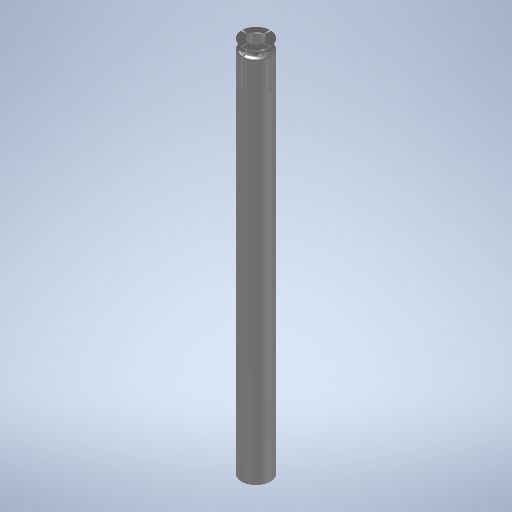
# Autodesk Inventor part: specimen_holder_rod_6mm
Saved by Autodesk Inventor 2023.2 (Build 272271000, 271)
## iProperties
Created: 2015-09-24
Part Number: specimen_holder_rod_6mm
Material: Edelstahl
Document SubType Name: Modeling
Designer: splath
Density: 8.08 g/cm^3
Appearance: Halbpoliert
Mass: 9.27092 g
Surface Area: 14.4867 cm^2
Volume: 1.14739 cm^3
Author: splath
Autodesk Inventor part; units mm, degrees
ref_plane "YZ Plane" through (0, 0, 0) normal (1, 0, 0) x (0, 1, 0)
ref_plane "XZ Plane" through (0, 0, 0) normal (0, 1, 0) x (-1, 0, 0)
sketch "Skizze1" plane through (0, 0, 0) normal (0, 0, 1) x (1, 0, 0)
  circle A0 centre (0, 0) radius 3
  dimension "d2" = 6
  constraints: 1 centre point, 1 coincident
  measures "d2" diameter of A0
extrude "Extrusion1" add sketch "Skizze1" against normal blind 70
sketch "Skizze2" plane through (0, 0, 0) normal (0, 0, 1) x (1, 0, 0)
  circle A0 centre (0, 0) radius 3 projected
  circle A1 centre (0, 0) radius 3
  dimension "d36" = 6
  constraints: 1 centre point, 1 coincident
  measures "d36" diameter of A1
extrude "Extrusion2" add sketch "Skizze2" along normal blind 1
sketch "Skizze3" plane through (0, 0, 1) normal (0, 0, 1) x (1, 0, 0)
  circle A0 centre (0, 0) radius 3 projected
  circle A1 centre (0, 0) radius 3
  dimension "d28" = 6
  constraints: 1 centre point, 1 coincident
  measures "d28" diameter of A1
extrude "Extrusion3" add sketch "Skizze3" along normal blind 8
ref_plane "Arbeitsebene1" through (0, 0, 2.5) normal (0, 0, 1) x (1, 0, 0)
sketch "Skizze4" plane through (0, 0, 2.5) normal (0, 0, 1) x (1, 0, 0)
  circle A0 centre (0, 0) radius 3
  constraints: 1 centre point, 1 coincident
extrude "Extrusion4" [suppressed]
hole "Bohrung1" at (0, 0, 9) direction (0, 0, -1) diameter 3 depth 23
chamfer "Fase1" distance 0.1 angle 45 1 edges at (0, 1.5, 9)
sketch "Skizze5" plane through (0, 0, 9) normal (0, 0, 1) x (1, 0, 0)
  circle A0 centre (0, 0) radius 3 projected
  line L0 (-3.5, -0.15) -> (3.5, -0.15)
  line L1 (3.5, -0.15) -> (3.5, 0.15)
  line L2 (3.5, 0.15) -> (-3.5, 0.15)
  line L3 (-3.5, 0.15) -> (-3.5, -0.15)
  line L4 (-3.5, -0.15) -> (3.5, 0.15) construction
  line L5 (3.5, -0.15) -> (-3.5, 0.15) construction
  line L6 (-0.15, -3.5) -> (0.15, -3.5)
  line L7 (0.15, -3.5) -> (0.15, 3.5)
  line L8 (0.15, 3.5) -> (-0.15, 3.5)
  line L9 (-0.15, 3.5) -> (-0.15, -3.5)
  line L10 (-0.15, -3.5) -> (0.15, 3.5) construction
  line L11 (0.15, -3.5) -> (-0.15, 3.5) construction
  constraints: 24 end point, 4 midpoint
extrude "Extrusion5" cut sketch "Skizze5" against normal up to surface (8 mm away) contours A0 L0 L7 L2 | A0 L2 L1 L0 | L7 L2 L9 A0 | A0 L9 L8 L7 | L7 L0 L9 L2 | L7 L6 L9 A0 | A0 L9 L0 L7 | L9 L0 A0 L2 | A0 L0 L3 L2
sketch "Skizze6" plane through (0, 0, 0) normal (0, 1, 0) x (-1, 0, 0)
  line L0 (0, 0) -> (-2, 0)
  line L1 (0, -1.8) -> (0, 10.8) projected
  circle A0 centre (-3, 8) radius 1
  line L2 (-0.15, 9) -> (-2.9962, 9) projected
  dimension "d33" = 3
  dimension "d34" = 2
  dimension "d35" = 1
  constraints: 2 end point, 1 centre point
  measures "d33" distance from line of L1 A0.centre
  measures "d34" diameter of A0
  measures "d35" distance from line of L2 A0.centre
revolve "Umdrehung1" cut sketch "Skizze6" angle 360 about axis through (0, 0, -10) along (0, 0, 1)
equation "\"d2\" = LowerDiameter"
equation "\"d0\" = LowerLength"
equation "\"d36\" = SealingRingDiameter"
equation "\"d3\" = SealingRingThickness"
equation "\"d28\" = UpperDiameter"
equation "\"d5\" = UpperLength"
equation "\"d9\" = DrillDiameter"
equation "\"d14\" = DrillDepth"
equation "\"UpperDiameter\" = 6"
equation "\"LowerDiameter\" = 6"
equation "\"UpperLength\" = 8"
equation "\"LowerLength\" = 70"
equation "\"SealingRingDiameter\" = 6"
equation "\"SealingRingThickness\" = 1"
equation "\"DrillDiameter\" = 3"
equation "\"DrillDepth\" = 23"
